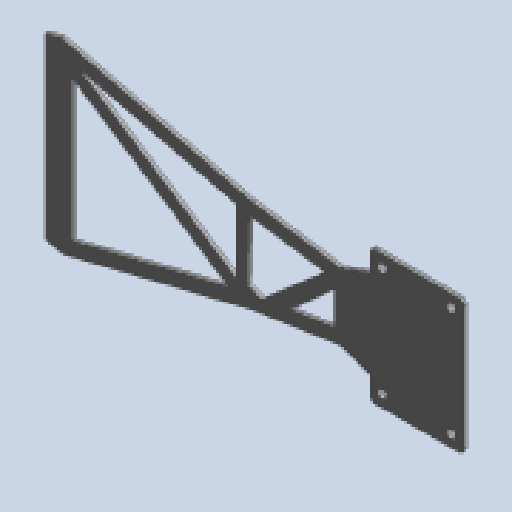
# Autodesk Inventor part: ShoulderMount
Saved by Autodesk Inventor 2023 (Build 270158000, 158)
## iProperties
Created: 2024-03-14
Part Number: ShoulderMount
Material: Generic
Document SubType Name: Sheet Metal
Designer: LattePanda
Density: 1 g/cm^3
Sheet Metal Rule: Default
Appearance: Default
Author: LattePanda
Autodesk Inventor part; units mm, degrees
ref_plane "YZ Plane" through (0, 0, 0) normal (1, 0, 0) x (0, 1, 0)
ref_plane "XZ Plane" through (0, 0, 0) normal (0, 1, 0) x (-1, 0, 0)
ref_plane "XY Plane" through (0, 0, 0) normal (0, 0, 1) x (1, 0, 0)
sketch "Mount" plane through (0, 0, 0) normal (0, 0, 1) x (1, 0, 0)
  circle A0 centre (-15.5, -1.5) radius 1.621 construction
  circle A1 centre (15.5, -1.5) radius 1.621 construction
  circle A2 centre (-15.5, -50.5) radius 1.621 construction
  circle A3 centre (15.5, -50.5) radius 1.621 construction
  line L0 (19, 6) -> (-19, 6) construction
  line L1 (19, -58) -> (-19, -58) construction
  circle A4 centre (-15.5, -1.5) radius 2
  circle A5 centre (15.5, -1.5) radius 2
  circle A6 centre (-15.5, -50.5) radius 2
  circle A7 centre (15.5, -50.5) radius 2
  line L2 (-21, 4) -> (21, 4)
  line L3 (21, 4) -> (21, -56)
  line L4 (21, -56) -> (-21, -56)
  line L5 (-21, -56) -> (-21, -46)
  line L6 (21, -51.5858) -> (21, -0.4142) construction
  line L7 (-21, 6) -> (-21, -6) construction
  line L8 (-19, -6) -> (19, -6) construction
  line L9 (-19, -46) -> (19, -46) construction
  line L10 (17, -8.5463) -> (13.9151, -6) construction
  line L11 (-17, -43.4537) -> (-13.9151, -46) construction
  line L12 (-21, -6) -> (-34, -11)
  line L13 (-21, -26) -> (-34, -26) construction
  line L14 (-34, -26) -> (-34, -11) construction
  line L15 (-21, -46) -> (-34, -41)
  line L16 (-34, -26) -> (-34, -41) construction
  line L17 (-74, -47) -> (-167.1457, 14) construction
  line L18 (-74, -47) -> (-74, -5) construction
  line L19 (-74, -5) -> (-159.3888, 15.957)
  line L20 (-159.3888, 15.957) -> (-167.1457, 14)
  line L21 (-167.1457, 14) -> (-167.1457, -26)
  line L22 (-167.1457, -26) -> (-74, -26) construction
  line L23 (-74, -47) -> (-159.3888, -67.957)
  line L24 (-159.3888, -67.957) -> (-167.1457, -66)
  line L25 (-167.1457, -66) -> (-167.1457, -26)
  line L26 (-34, -11) -> (-74, -5)
  line L27 (-34, -41) -> (-74, -47)
  line L28 (-74, -47) -> (-34, -11) construction
  line L29 (-34, -11) -> (21, -45.3945) construction
  line L30 (-151.8586, 7.9308) -> (-81.1625, -9.4202)
  line L31 (-81.1625, -9.4202) -> (-81.1625, -38.3672)
  line L32 (-81.1625, -38.3672) -> (-151.8586, 7.9308)
  line L33 (-41.0138, -16.0151) -> (-75.1625, -10.8927)
  line L34 (-155.1457, 2.9114) -> (-84.4497, -43.3866)
  line L35 (-84.4497, -43.3866) -> (-155.1457, -60.7376)
  line L36 (-155.1457, -60.7376) -> (-155.1457, 2.9114)
  line L37 (-56.8774, -38.3645) -> (-37, -20.4748)
  line L38 (-37, -20.4748) -> (-37, -35.3829)
  line L39 (-37, -35.3829) -> (-56.8774, -38.3645)
  line L40 (-155.1457, 2.9114) -> (-151.8586, 7.9308) construction
  line L41 (-81.1625, -38.3672) -> (-84.4497, -43.3866) construction
  line L42 (-37, -20.4748) -> (-41.0138, -16.0151) construction
  line L43 (-75.1625, -10.8927) -> (-76.1188, -38.3672)
  line L44 (-76.1188, -38.3672) -> (-69.5899, -40.779)
  line L45 (-69.5899, -40.779) -> (-41.0138, -16.0151)
  line L46 (-21, -6) -> (-21, 4)
  line L47 (-21, -46) -> (-21, -6) construction
  point P0 (0, 0)
  dimension "d0" = 4
  dimension "d1" = 4
  dimension "d2" = 4
  dimension "d3" = 4
  dimension "d7" = 2
  dimension "d8" = 2
  dimension "d15" = 80
  dimension "d16" = 8
  dimension "d17" = 13
  dimension "d18" = 40
  dimension "d19" = 93.1457
  dimension "d20" = 30
  dimension "d21" = 42
  dimension "d22" = 6
  dimension "d24" = 6
  dimension "d26" = 6
  dimension "d27" = 6
  dimension "d28" = 6
  dimension "d29" = 12
  dimension "d30" = 3
  measures "d0" diameter of A4
  measures "d1" diameter of A5
  measures "d2" diameter of A6
  measures "d3" diameter of A7
  measures "d8" distance between parallel lines of L1 L4
  measures "d15" distance of L25.start L17.end
  measures "d16" distance of L19.end L17.end
  measures "d17" distance between parallel lines of L5 L14
  measures "d18" distance between parallel lines of L14 L18
  measures "d19" distance between parallel lines of L18 L21
  measures "d20" distance of L15.end L12.end
  measures "d21" distance of L17.start L18.end
  measures "d22" distance between parallel lines of L19 L30
  measures "d24" distance between parallel lines of L26 L33
  measures "d26" distance between parallel lines of L27 L39
  measures "d27" distance between parallel lines of L23 L35
  measures "d28" distance between parallel lines of L34 L32
  measures "d29" distance between parallel lines of L21 L36
  measures "d30" distance between parallel lines of L14 L38
extrude "Plate1" add sketch "Mount" along normal blind 1.6002
fillet "MountFilletsFeature" radius 2 4 edges at (21, 4, 0.8001) (-21, 4, 0.8001) (21, -56, 0.8001) (-21, -56, 0.8001)
equation "\"d24\" = d22"
equation "\"d26\" = d22"
equation "\"d27\" = d22"
equation "\"d28\" = d22"
equation "\"d29\" = 2 * d22"
equation "\"d30\" = 0.5 * d22"
equation "\"d9\" = Thickness"
equation "\"BendRadius\" = Thickness"
equation "\"BendReliefWidth\" = Thickness"
equation "\"BendReliefDepth\" = 0.5 * Thickness"
equation "\"CornerReliefSize\" = 4 * Thickness"
equation "\"MinimumRemnant\" = 2 * Thickness"
equation "\"TransitionRadius\" = BendRadius"
equation "\"JacobiRadiusSize\" = BendRadius"
equation "\"GapSize\" = Thickness"
equation "\"Thickness\" = 1.6002"
body "Solid1"
